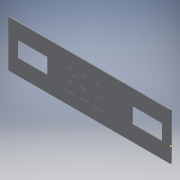
# Autodesk Inventor part: upper Ramp
Saved by Autodesk Inventor 2018.2 (Build 222227000, 227)
## iProperties
Created: 2018-02-11
Part Number: upper Ramp
Material: Generic
Document SubType Name: Modeling
Designer: Orangeracer
Density: 1 g/cm^3
Appearance: Default
Author: Orangeracer
Autodesk Inventor part; units mm, degrees
ref_plane "YZ Plane" through (0, 0, 0) normal (1, 0, 0) x (0, 1, 0)
ref_plane "XZ Plane" through (0, 0, 0) normal (0, 1, 0) x (-1, 0, 0)
ref_plane "XY Plane" through (0, 0, 0) normal (0, 0, 1) x (1, 0, 0)
sketch "Sketch1" plane through (0, 0, 0) normal (0, 0, 1) x (1, 0, 0)
  line L0 (0, 0) -> (-530.225, 0)
  line L1 (-530.225, 0) -> (-530.225, -50.8)
  line L2 (-530.225, -50.8) -> (0, -50.8)
  line L3 (0, -50.8) -> (0, 0)
  line L4 (-403.225, 0) -> (-127, 0)
  line L5 (-127, 0) -> (-127, 50.8)
  line L6 (-127, 50.8) -> (-403.225, 50.8)
  line L7 (-403.225, 50.8) -> (-403.225, 0)
  line L8 (0, 50.8) -> (-530.225, 50.8)
  line L9 (-530.225, 50.8) -> (-530.225, 101.6)
  line L10 (-530.225, 101.6) -> (0, 101.6)
  line L11 (0, 101.6) -> (0, 50.8)
  line L12 (-530.225, 0) -> (-501.65, 0)
  line L13 (-501.65, 0) -> (-501.65, 50.8)
  line L14 (-501.65, 50.8) -> (-530.225, 50.8)
  line L15 (-530.225, 50.8) -> (-530.225, 0)
  line L16 (0, 0) -> (-28.575, 0)
  line L17 (-28.575, 0) -> (-28.575, 50.8)
  line L18 (-28.575, 50.8) -> (0, 50.8)
  line L19 (0, 50.8) -> (0, 0)
  dimension "d0" = 530.225
  dimension "d1" = 50.8
  dimension "d2" = 50.8
  dimension "d3" = 127
  dimension "d4" = 127
  dimension "d5" = 50.8
  dimension "d6" = 530.225
  dimension "d7" = 0
  dimension "d8" = 50.8
  dimension "d9" = 28.575
  dimension "d10" = 28.575
  constraints: 40 end point, 10 parallel, 5 horizontal, 5 perpendicular, 3 point on line
  measures "d0" distance of L2.end L1.end
  measures "d1" distance of L1.end L0.end
  measures "d2" distance of L4.end L5.end
  measures "d3" distance between parallel lines of L3 L5
  measures "d4" distance between parallel lines of L1 L7
  measures "d5" distance of L8.end L9.end
  measures "d6" distance of L9.end L10.end
  measures "d7" distance between parallel lines of L3 L11
  measures "d8" distance between parallel lines of L8 L0
  measures "d9" distance of L14.end L13.end
  measures "d10" distance of L17.end L18.end
extrude "Extrusion1" add sketch "Sketch1" along normal blind 3.175 contours L3 L2 L1 L0 | L0 L17 L8 L19 | L8 L6 L9 L10 L11 | L0 L7 L6 L5 | L15 L8 L13 L0
sketch "Sketch2" plane through (0, 0, 3.175) normal (0, 0, 1) x (1, 0, 0)
  line L0 (-352.425, 63.5) -> (-177.8, 63.5) construction
  line L1 (-177.8, 63.5) -> (-177.8, -1.2974) construction
  line L2 (-177.8, -1.2974) -> (-352.425, -1.2974) construction
  line L3 (-352.425, -1.2974) -> (-352.425, 63.5) construction
  line L4 (-403.225, 50.8) -> (-403.225, 0) projected
  line L5 (-127, 0) -> (-127, 50.8) projected
  line L6 (0, 101.6) -> (-530.225, 101.6) projected
  spline S0 degree 2 poles (-311.0058, -6.6857) (-311.0058, -12.7) (-317.0201, -12.7) knots 0 0 0 1 1 1
  line L7 (-317.0201, -12.7) -> (-341.8149, -12.7)
  spline S1 degree 2 poles (-341.8149, -12.7) (-347.8292, -12.7) (-347.8292, -6.6857) knots 0 0 0 1 1 1
  line L8 (-347.8292, -6.6857) -> (-347.8292, 57.4857)
  spline S2 degree 2 poles (-347.8292, 57.4857) (-347.8292, 63.5) (-341.9284, 63.5) knots 0 0 0 1 1 1
  line L9 (-341.9284, 63.5) -> (-317.247, 63.5)
  spline S3 degree 2 poles (-317.247, 63.5) (-311.176, 63.5) (-311.176, 57.4857) knots 0 0 0 1 1 1
  line L10 (-311.176, 57.4857) -> (-311.176, 40.4074)
  line L11 (-311.176, 40.4074) -> (-322.3535, 40.4074)
  line L12 (-322.3535, 40.4074) -> (-322.3535, 53.741)
  line L13 (-322.3535, 53.741) -> (-336.6517, 53.741)
  line L14 (-336.6517, 53.741) -> (-336.6517, 30.8185)
  line L15 (-336.6517, 30.8185) -> (-317.0201, 30.8185)
  spline S4 degree 2 poles (-317.0201, 30.8185) (-311.0058, 30.8185) (-311.0058, 24.8042) knots 0 0 0 1 1 1
  line L16 (-311.0058, 24.8042) -> (-311.0058, -6.6857)
  line L17 (-322.1266, -2.941) -> (-322.1266, 21.1162)
  line L18 (-322.1266, 21.1162) -> (-336.6517, 21.1162)
  line L19 (-336.6517, 21.1162) -> (-336.6517, -2.941)
  line L20 (-336.6517, -2.941) -> (-322.1266, -2.941)
  spline S5 degree 2 poles (-265.161, -6.6857) (-265.161, -12.7) (-271.1753, -12.7) knots 0 0 0 1 1 1
  line L21 (-271.1753, -12.7) -> (-296.0835, -12.7)
  spline S6 degree 2 poles (-296.0835, -12.7) (-301.8141, -12.7) (-301.8141, -6.6857) knots 0 0 0 1 1 1
  line L22 (-301.8141, -6.6857) -> (-301.8141, 10.3926)
  line L23 (-301.8141, 10.3926) -> (-290.6366, 10.3926)
  line L24 (-290.6366, 10.3926) -> (-290.6366, -2.941)
  line L25 (-290.6366, -2.941) -> (-276.452, -2.941)
  line L26 (-276.452, -2.941) -> (-276.452, 19.9815)
  line L27 (-276.452, 19.9815) -> (-296.4807, 19.9815)
  spline S7 degree 2 poles (-296.4807, 19.9815) (-302.0978, 19.9815) (-302.0978, 25.9958) knots 0 0 0 1 1 1
  line L28 (-302.0978, 25.9958) -> (-302.0978, 57.4857)
  spline S8 degree 2 poles (-302.0978, 57.4857) (-302.0978, 63.5) (-296.4807, 63.5) knots 0 0 0 1 1 1
  line L29 (-296.4807, 63.5) -> (-271.2887, 63.5)
  spline S9 degree 2 poles (-271.2887, 63.5) (-265.161, 63.5) (-265.161, 57.4857) knots 0 0 0 1 1 1
  line L30 (-265.161, 57.4857) -> (-265.161, -6.6857)
  line L31 (-276.452, 29.627) -> (-276.452, 53.741)
  line L32 (-276.452, 53.741) -> (-290.977, 53.741)
  line L33 (-290.977, 53.741) -> (-290.977, 29.627)
  line L34 (-290.977, 29.627) -> (-276.452, 29.627)
  spline S10 degree 2 poles (-218.3516, -6.6857) (-218.3516, -12.7) (-224.3659, -12.7) knots 0 0 0 1 1 1
  line L35 (-224.3659, -12.7) -> (-250.0117, -12.7)
  spline S11 degree 2 poles (-250.0117, -12.7) (-256.026, -12.7) (-256.026, -6.6857) knots 0 0 0 1 1 1
  line L36 (-256.026, -6.6857) -> (-256.026, 16.4069)
  spline S12 degree 2 poles (-256.026, 16.4069) (-256.026, 20.6056) (-253.1891, 22.8751) knots 0 0 0 1 1 1
  spline S13 degree 2 poles (-253.1891, 22.8751) (-249.8415, 24.8042) (-246.4372, 26.7901) knots 0 0 0 1 1 1
  spline S14 degree 2 poles (-246.4372, 26.7901) (-249.7281, 28.6625) (-252.9622, 30.5916) knots 0 0 0 1 1 1
  spline S15 degree 2 poles (-252.9622, 30.5916) (-255.9126, 32.9179) (-255.9126, 36.8896) knots 0 0 0 1 1 1
  line L37 (-255.9126, 36.8896) -> (-255.9126, 57.4857)
  spline S16 degree 2 poles (-255.9126, 57.4857) (-255.9126, 63.5) (-249.7281, 63.5) knots 0 0 0 1 1 1
  line L38 (-249.7281, 63.5) -> (-224.4794, 63.5)
  spline S17 degree 2 poles (-224.4794, 63.5) (-218.5218, 63.5) (-218.5218, 57.4857) knots 0 0 0 1 1 1
  line L39 (-218.5218, 57.4857) -> (-218.5218, 36.8896)
  spline S18 degree 2 poles (-218.5218, 36.8896) (-218.5218, 32.8611) (-221.4722, 30.5916) knots 0 0 0 1 1 1
  spline S19 degree 2 poles (-221.4722, 30.5916) (-224.7063, 28.6625) (-227.9972, 26.7901) knots 0 0 0 1 1 1
  spline S20 degree 2 poles (-227.9972, 26.7901) (-224.6496, 24.8042) (-221.2453, 22.8751) knots 0 0 0 1 1 1
  spline S21 degree 2 poles (-221.2453, 22.8751) (-218.3516, 20.6056) (-218.3516, 16.4069) knots 0 0 0 1 1 1
  line L40 (-218.3516, 16.4069) -> (-218.3516, -6.6857)
  line L41 (-229.6993, -3.1112) -> (-229.6993, 17.9956)
  line L42 (-229.6993, 17.9956) -> (-237.1888, 22.3077)
  line L43 (-237.1888, 22.3077) -> (-244.7351, 17.9956)
  line L44 (-244.7351, 17.9956) -> (-244.7351, -3.1112)
  line L45 (-244.7351, -3.1112) -> (-229.6993, -3.1112)
  line L46 (-229.8128, 35.6413) -> (-229.8128, 53.9112)
  line L47 (-229.8128, 53.9112) -> (-244.5648, 53.9112)
  line L48 (-244.5648, 53.9112) -> (-244.5648, 35.6413)
  line L49 (-244.5648, 35.6413) -> (-237.1888, 31.2725)
  line L50 (-237.1888, 31.2725) -> (-229.8128, 35.6413)
  point P0 (0, 0)
  dimension "d13" = 50.8
  dimension "d14" = 50.8
  dimension "d15" = 38.1
  constraints: 2 other
  measures "d13" distance between parallel lines of L4 L3
  measures "d14" distance between parallel lines of L5 L1
  measures "d15" distance between parallel lines of L6 L0
extrude "Extrusion2" cut sketch "Sketch2" against normal blind 0.7937
sketch "Sketch3" plane through (0, 0, 3.175) normal (0, 0, 1) x (1, 0, 0)
  point P0 (0, 0)
body "Solid1"
